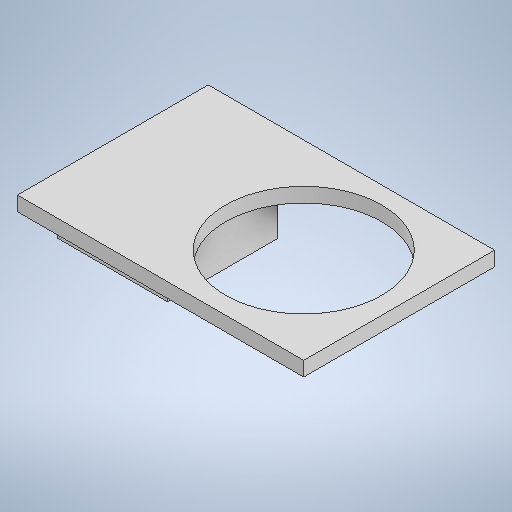
# Autodesk Inventor part: joystick_test_v3
Saved by Autodesk Inventor 2025.4 (Build 294407000, 407)
## iProperties
Created: 2026-07-26
Part Number: joystick_test_v3
Material: Generic
Document SubType Name: Modeling
Designer: Franchesca
Density: 1 g/cm^3
Appearance: Default
Author: Franchesca
## iProperties of the stored document joystick_test_v2_3DPrint.ipt
Created: 2026-07-26
Part Number: joystick_test_v2_3DPrint
Material: Generic
Document SubType Name: Modeling
Designer: Franchesca
Density: 1 g/cm^3
Appearance: Default
Author: Franchesca
Autodesk Inventor part; units mm, degrees
ref_plane "YZ Plane" through (0, 0, 0) normal (1, 0, 0) x (0, 1, 0)
ref_plane "XZ Plane" through (0, 0, 0) normal (0, 1, 0) x (-1, 0, 0)
ref_plane "XY Plane" through (0, 0, 0) normal (0, 0, 1) x (1, 0, 0)
sketch "Sketch1" plane through (0, 0, 0) normal (0, 1, 0) x (-1, 0, 0)
  circle A0 centre (0, 0) radius 13.5
  line L0 (0, -13.5) -> (30, -13.5) construction
  line L1 (0, 13.5) -> (30, 13.5) construction
  line L2 (30, 13.5) -> (30, -13.5) construction
  line L3 (0, -13.5) -> (16, -13.5) construction
  line L4 (0, 13.5) -> (16, 13.5) construction
  line L5 (16, 13.5) -> (16, -13.5) construction
  line L6 (30, 13.5) -> (30, 9.5) construction
  line L7 (30, -13.5) -> (30, -9.5) construction
  line L8 (0, -13.5) -> (0, -16.5) construction
  line L9 (0, 13.5) -> (0, 16.5) construction
  line L10 (30, -2.5) -> (33, -2.5) construction
  line L11 (-13.5, 0) -> (-16.5, 0) construction
  line L12 (33, -2.5) -> (33, -16.5)
  line L13 (33, -16.5) -> (0, -16.5)
  line L14 (33, -2.5) -> (33, 16.5)
  line L15 (33, 16.5) -> (0, 16.5)
  line L16 (0, 16.5) -> (-16.5, 16.5)
  line L17 (-16.5, 0) -> (-16.5, 16.5)
  line L18 (0, -16.5) -> (-16.5, -16.5)
  line L19 (-16.5, -16.5) -> (-16.5, 0)
  line L20 (0, 13.5) -> (14, 13.5) construction
  line L21 (0, -13.5) -> (14, -13.5) construction
  line L22 (14, 13.5) -> (14, -13.5) construction
  line L23 (33, 9.5) -> (33, 10.5) construction
  line L24 (33, -9.5) -> (33, -10.5) construction
  line L25 (14, -11.5) -> (14, -6.5) construction
  line L26 (14, 10.5) -> (14, 5.5) construction
  line L27 (0, -13.5) -> (15, -13.5) construction
  line L28 (0, 13.5) -> (15, 13.5) construction
  line L29 (15, 13.5) -> (15, -13.5) construction
  line L30 (14, -11.5) -> (14, -6.5) construction
  line L31 (14, -13.5) -> (14, -8.5) construction
  line L32 (14, 13.5) -> (14, 8.5) construction
  line L33 (14, 8.5) -> (30, 8.5) construction
  line L34 (14, -8.5) -> (30, -8.5) construction
  line L35 (16, -8.5) -> (16, -9.5) construction
  line L36 (16, 8.5) -> (16, 9.5) construction
  line L37 (16, 8.5) -> (16, 7.5) construction
  line L38 (16, -8.5) -> (16, -7.5) construction
  line L39 (30, -9.5) -> (14, -9.5) construction
  line L40 (30, 9.5) -> (14, 9.5) construction
  line L41 (14, -9.5) -> (33, -9.5)
  line L42 (14, 9.5) -> (33, 9.5)
  line L43 (33, 8.5) -> (15, 8.5)
  line L44 (15, 8.5) -> (15, -8.5)
  line L45 (15, -8.5) -> (33, -8.5)
  line L46 (14, -9.5) -> (14, 9.5)
  line L47 (33, -9.5) -> (33, 8.5)
  dimension "d0" = 27
  dimension "d1" = 30
  dimension "d2" = 30
  dimension "d3" = 16
  dimension "d4" = 16
  dimension "d5" = 4
  dimension "d6" = 4
  dimension "d7" = 3
  dimension "d8" = 3
  dimension "d9" = 3
  dimension "d10" = 3
  dimension "d16" = 14
  dimension "d17" = 14
  dimension "d26" = 15
  dimension "d27" = 15
  dimension "d29" = 5
  dimension "d30" = 5
  dimension "d31" = 1
  dimension "d32" = 1
  dimension "d33" = 1
  dimension "d34" = 1
  constraints: 96 end point, 38 point on line, 11 perpendicular, 4 horizontal, 4 vertical, 3 collinear, 3 point on circle, 2 tangent, 1 centre point, 1 coincident, 1 midpoint
  measures "d0" diameter of A0
  measures "d1" distance of L0.start L0.end
  measures "d2" distance of L1.start L1.end
  measures "d3" distance of L0.start L3.end
  measures "d4" distance of L1.start L4.end
  measures "d5" distance of L1.end L6.end
  measures "d6" distance of L0.end L7.end
  measures "d7" distance of L0.start L8.end
  measures "d8" distance of L1.start L9.end
  measures "d9" distance of L10.start L10.end
  measures "d10" distance of L11.start L11.end
  measures "d16" distance of L1.start L20.end
  measures "d17" distance of L0.start L21.end
  measures "d26" distance of L0.start L27.end
  measures "d27" distance of L1.start L28.end
  measures "d29" distance of L21.end L31.end
  measures "d30" distance of L20.end L32.end
  measures "d31" distance of L35.start L35.end
  measures "d32" distance of L36.start L36.end
  measures "d33" distance of L36.start L37.end
  measures "d34" distance of L35.start L38.end
extrude "Extrusion5" add sketch "Sketch1" against normal blind 2.5 contours L12 L13 L18 L19 L17 L16 L15 L14 L42 L46 L41
extrude "Extrusion6" add sketch "Sketch1" against normal blind 10 contours L12 L41 L46 L42 L14 L43 L44 L45
extrude "Extrusion7" add sketch "Sketch1" against normal blind 4 contours L12 L45 L44 L43 L14
body "Solid3"
